Autodesk Inventor part; units mm, degrees
(part 2 of 3)
  spline S35 degree 3 poles (-630.6754, -331.5189) (-629.2902, -331.389) (-626.5198, -331.1292) (-622.3727, -330.655) (-618.2337, -330.1163) (-614.104, -329.509) (-609.9888, -328.8126) (-606.9048, -328.2722) (-604.8663, -327.8241) (-603.9999, -327.726) (-603.303, -327.7315) (-602.786, -327.8061) (-602.2738, -327.9106) (-601.7834, -328.092) (-601.3076, -328.3077) (-600.7153, -328.6749) (-600.1921, -329.1421) (-599.7524, -329.6826) (-599.3924, -330.2793) (-598.9871, -331.0485) (-598.5515, -331.8009) (-598.2378, -332.4231) (-598.014, -333.083) (-597.8968, -333.7746) (-597.901, -334.4715) (-597.9715, -334.9891) (-598.0788, -335.5008) (-598.2628, -335.9901) (-598.4747, -336.4676) (-598.8409, -337.0606) (-599.3849, -337.742) (-600.8488, -339.2296) (-602.9472, -341.5534) (-605.7262, -344.6674) (-608.4377, -347.841) (-611.0958, -351.059) (-613.7038, -354.3181) (-615.3977, -356.5256) (-616.2446, -357.6294) knots 0 0 0 0 0.062506 0.125011 0.187517 0.250023 0.312528 0.375034 0.390661 0.406272 0.414085 0.421898 0.429707 0.43752 0.44533 0.453144 0.468748 0.476562 0.484374 0.5 0.515626 0.523438 0.531252 0.546856 0.55467 0.56248 0.570293 0.578102 0.585915 0.593728 0.609339 0.624966 0.687472 0.749977 0.812483 0.874989 0.937494 1 1 1 1 projected
  arc A39 (-616.2446, -357.6294) -> (-611.0948, -366.3596) centre (0, 0) ccw projected
  spline S36 degree 3 poles (-611.0948, -366.3596) (-609.7191, -366.1523) (-606.9676, -365.7376) (-602.8536, -365.0315) (-598.7514, -364.2616) (-594.6622, -363.4237) (-590.5925, -362.4976) (-587.5436, -361.7852) (-585.5335, -361.2235) (-584.674, -361.077) (-583.9779, -361.0434) (-583.4575, -361.0889) (-582.9402, -361.1645) (-582.4404, -361.3181) (-581.9532, -361.5068) (-581.3414, -361.8402) (-580.7927, -362.2774) (-580.3234, -362.7924) (-579.9306, -363.3679) (-579.4827, -364.1131) (-579.0056, -364.8399) (-578.6575, -365.4436) (-578.3971, -366.0899) (-578.2414, -366.7739) (-578.2064, -367.4699) (-578.2478, -367.9906) (-578.3263, -368.5076) (-578.4825, -369.0064) (-578.6673, -369.495) (-578.9997, -370.1076) (-579.5046, -370.8184) (-580.8828, -372.3858) (-582.8476, -374.8236) (-585.4477, -378.0885) (-587.9769, -381.4091) (-590.4504, -384.7711) (-592.8715, -388.1713) (-594.439, -390.4704) (-595.2227, -391.6199) knots 0 0 0 0 0.062506 0.125011 0.187517 0.250023 0.312528 0.375034 0.390661 0.406272 0.414085 0.421898 0.429707 0.43752 0.44533 0.453144 0.468748 0.476562 0.484374 0.5 0.515626 0.523438 0.531252 0.546856 0.55467 0.56248 0.570293 0.578102 0.585915 0.593728 0.609339 0.624966 0.687472 0.749977 0.812483 0.874989 0.937494 1 1 1 1 projected
  arc A40 (-595.2227, -391.6199) -> (-589.5915, -400.0476) centre (0, 0) ccw projected
  spline S37 degree 3 poles (-589.5915, -400.0476) (-588.2295, -399.7635) (-585.5056, -399.1951) (-581.4377, -398.2595) (-577.3851, -397.2608) (-573.3493, -396.1949) (-569.338, -395.0422) (-566.3339, -394.1599) (-564.3583, -393.4864) (-563.5084, -393.2919) (-562.8153, -393.2193) (-562.2931, -393.2355) (-561.7725, -393.2821) (-561.2648, -393.4074) (-560.7679, -393.5684) (-560.1383, -393.8671) (-559.566, -394.2727) (-559.0685, -394.7606) (-558.644, -395.3133) (-558.1551, -396.0322) (-557.638, -396.7311) (-557.2566, -397.3143) (-556.9604, -397.945) (-556.7665, -398.6191) (-556.6926, -399.312) (-556.7047, -399.8343) (-556.7541, -400.3549) (-556.8821, -400.8617) (-557.0392, -401.3599) (-557.3367, -401.9901) (-557.801, -402.7281) (-559.0892, -404.3703) (-560.9141, -406.9145) (-563.327, -410.32) (-565.6661, -413.7772) (-567.9472, -417.2726) (-570.1739, -420.8032) (-571.61, -423.1866) (-572.328, -424.3782) knots 0 0 0 0 0.062506 0.125011 0.187517 0.250023 0.312528 0.375034 0.390661 0.406272 0.414085 0.421898 0.429707 0.43752 0.44533 0.453144 0.468748 0.476562 0.484374 0.5 0.515626 0.523438 0.531252 0.546856 0.55467 0.56248 0.570293 0.578102 0.585915 0.593728 0.609339 0.624966 0.687472 0.749977 0.812483 0.874989 0.937494 1 1 1 1 projected
  arc A41 (-572.328, -424.3782) -> (-566.2331, -432.4769) centre (0, 0) ccw projected
  spline S38 degree 3 poles (-566.2331, -432.4769) (-564.8892, -432.1169) (-562.2015, -431.3967) (-558.1924, -430.2345) (-554.2022, -429.0101) (-550.2325, -427.7196) (-546.2921, -426.3437) (-543.3422, -425.2944) (-541.4076, -424.5112) (-540.5699, -424.2693) (-539.8819, -424.158) (-539.3597, -424.1449) (-538.8372, -424.1622) (-538.3233, -424.2589) (-537.8181, -424.3918) (-537.1728, -424.6546) (-536.5786, -425.0276) (-536.0546, -425.4868) (-535.5998, -426.0148) (-535.0713, -426.7051) (-534.5159, -427.374) (-534.1023, -427.9349) (-533.7712, -428.5479) (-533.5398, -429.2102) (-533.4272, -429.8979) (-533.41, -430.42) (-533.4301, -430.9425) (-533.5296, -431.4557) (-533.6585, -431.9619) (-533.9201, -432.6078) (-534.3423, -433.3707) (-535.5364, -435.0826) (-537.2158, -437.725) (-539.434, -441.2605) (-541.5755, -444.8434) (-543.6571, -448.4612) (-545.6823, -452.1111) (-546.9825, -454.5712) (-547.6326, -455.8013) knots 0 0 0 0 0.062506 0.125011 0.187517 0.250023 0.312528 0.375034 0.390661 0.406272 0.414085 0.421898 0.429707 0.43752 0.44533 0.453144 0.468748 0.476562 0.484374 0.5 0.515626 0.523438 0.531252 0.546856 0.55467 0.56248 0.570293 0.578102 0.585915 0.593728 0.609339 0.624966 0.687472 0.749977 0.812483 0.874989 0.937494 1 1 1 1 projected
  arc A42 (-547.6326, -455.8013) -> (-541.0931, -463.5455) centre (0, 0) ccw projected
  spline S39 degree 3 poles (-541.0931, -463.5455) (-539.7716, -463.1107) (-537.1284, -462.2409) (-533.1909, -460.8557) (-529.2755, -459.4096) (-525.3845, -457.8985) (-521.5274, -456.3038) (-518.641, -455.0908) (-516.7533, -454.2003) (-515.9305, -453.9119) (-515.2498, -453.7621) (-514.7292, -453.7198) (-514.2066, -453.7077) (-513.6881, -453.7755) (-513.1762, -453.8798) (-512.5171, -454.1061) (-511.903, -454.4451) (-511.354, -454.8742) (-510.8703, -455.3759) (-510.304, -456.0355) (-509.7119, -456.6722) (-509.2676, -457.209) (-508.9026, -457.8025) (-508.6345, -458.4508) (-508.4834, -459.131) (-508.4371, -459.6514) (-508.4278, -460.1742) (-508.4983, -460.6921) (-508.5986, -461.2048) (-508.8237, -461.8644) (-509.2024, -462.6498) (-510.2986, -464.4259) (-511.8272, -467.1583) (-513.8437, -470.8126) (-515.781, -474.51) (-517.6564, -478.2388) (-519.4737, -481.9965) (-520.634, -484.5257) (-521.2141, -485.7902) knots 0 0 0 0 0.062506 0.125011 0.187517 0.250023 0.312528 0.375034 0.390661 0.406272 0.414085 0.421898 0.429707 0.43752 0.44533 0.453144 0.468748 0.476562 0.484374 0.5 0.515626 0.523438 0.531252 0.546856 0.55467 0.56248 0.570293 0.578102 0.585915 0.593728 0.609339 0.624966 0.687472 0.749977 0.812483 0.874989 0.937494 1 1 1 1 projected
  arc A43 (-521.2141, -485.7902) -> (-514.2507, -493.1556) centre (0, 0) ccw projected
  spline S40 degree 3 poles (-514.2507, -493.1556) (-512.9556, -492.6473) (-510.3654, -491.6307) (-506.5117, -490.027) (-502.6836, -488.3636) (-498.8834, -486.6367) (-495.1218, -484.8283) (-492.3079, -483.4553) (-490.4731, -482.4603) (-489.6678, -482.1262) (-488.9966, -481.9385) (-488.4791, -481.8671) (-487.958, -481.8258) (-487.4366, -481.8643) (-486.9196, -481.9398) (-486.2489, -482.1288) (-485.6167, -482.4328) (-485.0446, -482.8305) (-484.5335, -483.3042) (-483.9311, -483.9311) (-483.3042, -484.5335) (-482.8305, -485.0446) (-482.4328, -485.6167) (-482.1288, -486.2489) (-481.9398, -486.9196) (-481.8643, -487.4366) (-481.8258, -487.958) (-481.8671, -488.4791) (-481.9385, -488.9966) (-482.1262, -489.6678) (-482.4603, -490.4731) (-483.4553, -492.3079) (-484.8283, -495.1218) (-486.6367, -498.8834) (-488.3636, -502.6836) (-490.027, -506.5117) (-491.6307, -510.3654) (-492.6473, -512.9556) (-493.1556, -514.2507) knots 0 0 0 0 0.062506 0.125011 0.187517 0.250023 0.312528 0.375034 0.390661 0.406272 0.414085 0.421898 0.429707 0.43752 0.44533 0.453144 0.468748 0.476562 0.484374 0.5 0.515626 0.523438 0.531252 0.546856 0.55467 0.56248 0.570293 0.578102 0.585915 0.593728 0.609339 0.624966 0.687472 0.749977 0.812483 0.874989 0.937494 1 1 1 1 projected
  arc A44 (-493.1556, -514.2507) -> (-485.7902, -521.2141) centre (0, 0) ccw projected
  spline S41 degree 3 poles (-485.7902, -521.2141) (-484.5257, -520.634) (-481.9965, -519.4737) (-478.2388, -517.6564) (-474.51, -515.781) (-470.8126, -513.8437) (-467.1583, -511.8272) (-464.4259, -510.2986) (-462.6498, -509.2024) (-461.8644, -508.8237) (-461.2048, -508.5986) (-460.6921, -508.4983) (-460.1742, -508.4278) (-459.6514, -508.4371) (-459.131, -508.4834) (-458.4508, -508.6345) (-457.8025, -508.9026) (-457.209, -509.2676) (-456.6722, -509.7119) (-456.0355, -510.304) (-455.3759, -510.8703) (-454.8742, -511.354) (-454.4451, -511.903) (-454.1061, -512.5171) (-453.8798, -513.1762) (-453.7755, -513.6881) (-453.7077, -514.2066) (-453.7198, -514.7292) (-453.7621, -515.2498) (-453.9119, -515.9305) (-454.2003, -516.7533) (-455.0908, -518.641) (-456.3038, -521.5274) (-457.8985, -525.3845) (-459.4096, -529.2755) (-460.8557, -533.1909) (-462.2409, -537.1284) (-463.1107, -539.7716) (-463.5455, -541.0931) knots 0 0 0 0 0.062506 0.125011 0.187517 0.250023 0.312528 0.375034 0.390661 0.406272 0.414085 0.421898 0.429707 0.43752 0.44533 0.453144 0.468748 0.476562 0.484374 0.5 0.515626 0.523438 0.531252 0.546856 0.55467 0.56248 0.570293 0.578102 0.585915 0.593728 0.609339 0.624966 0.687472 0.749977 0.812483 0.874989 0.937494 1 1 1 1 projected
  arc A45 (-463.5455, -541.0931) -> (-455.8013, -547.6326) centre (0, 0) ccw projected
  spline S42 degree 3 poles (-455.8013, -547.6326) (-454.5712, -546.9825) (-452.1111, -545.6823) (-448.4612, -543.6571) (-444.8434, -541.5755) (-441.2605, -539.434) (-437.725, -537.2158) (-435.0826, -535.5364) (-433.3707, -534.3423) (-432.6078, -533.9201) (-431.9619, -533.6585) (-431.4557, -533.5296) (-430.9425, -533.4301) (-430.42, -533.41) (-429.8979, -533.4272) (-429.2102, -533.5398) (-428.5479, -533.7712) (-427.9349, -534.1023) (-427.374, -534.5159) (-426.7051, -535.0713) (-426.0148, -535.5998) (-425.4868, -536.0546) (-425.0276, -536.5786) (-424.6546, -537.1728) (-424.3918, -537.8181) (-424.2589, -538.3233) (-424.1622, -538.8372) (-424.1449, -539.3597) (-424.158, -539.8819) (-424.2693, -540.5699) (-424.5112, -541.4076) (-425.2944, -543.3422) (-426.3437, -546.2921) (-427.7196, -550.2325) (-429.0101, -554.2022) (-430.2345, -558.1924) (-431.3967, -562.2015) (-432.1169, -564.8892) (-432.4769, -566.2331) knots 0 0 0 0 0.062506 0.125011 0.187517 0.250023 0.312528 0.375034 0.390661 0.406272 0.414085 0.421898 0.429707 0.43752 0.44533 0.453144 0.468748 0.476562 0.484374 0.5 0.515626 0.523438 0.531252 0.546856 0.55467 0.56248 0.570293 0.578102 0.585915 0.593728 0.609339 0.624966 0.687472 0.749977 0.812483 0.874989 0.937494 1 1 1 1 projected
  arc A46 (-432.4769, -566.2331) -> (-424.3782, -572.328) centre (0, 0) ccw projected
  spline S43 degree 3 poles (-424.3782, -572.328) (-423.1866, -571.61) (-420.8032, -570.1739) (-417.2726, -567.9472) (-413.7772, -565.6661) (-410.32, -563.327) (-406.9145, -560.9141) (-404.3703, -559.0892) (-402.7281, -557.801) (-401.9901, -557.3367) (-401.3599, -557.0392) (-400.8617, -556.8821) (-400.3549, -556.7541) (-399.8343, -556.7047) (-399.312, -556.6926) (-398.6191, -556.7665) (-397.945, -556.9604) (-397.3143, -557.2566) (-396.7311, -557.638) (-396.0322, -558.1551) (-395.3133, -558.644) (-394.7606, -559.0685) (-394.2727, -559.566) (-393.8671, -560.1383) (-393.5684, -560.7679) (-393.4074, -561.2648) (-393.2821, -561.7725) (-393.2355, -562.2931) (-393.2193, -562.8153) (-393.2919, -563.5084) (-393.4864, -564.3583) (-394.1599, -566.3339) (-395.0422, -569.338) (-396.1949, -573.3493) (-397.2608, -577.3851) (-398.2595, -581.4377) (-399.1951, -585.5056) (-399.7635, -588.2295) (-400.0476, -589.5915) knots 0 0 0 0 0.062506 0.125011 0.187517 0.250023 0.312528 0.375034 0.390661 0.406272 0.414085 0.421898 0.429707 0.43752 0.44533 0.453144 0.468748 0.476562 0.484374 0.5 0.515626 0.523438 0.531252 0.546856 0.55467 0.56248 0.570293 0.578102 0.585915 0.593728 0.609339 0.624966 0.687472 0.749977 0.812483 0.874989 0.937494 1 1 1 1 projected
  arc A47 (-400.0476, -589.5915) -> (-391.6199, -595.2227) centre (0, 0) ccw projected
  spline S44 degree 3 poles (-391.6199, -595.2227) (-390.4704, -594.439) (-388.1713, -592.8715) (-384.7711, -590.4504) (-381.4091, -587.9769) (-378.0885, -585.4477) (-374.8236, -582.8476) (-372.3858, -580.8828) (-370.8184, -579.5046) (-370.1076, -578.9997) (-369.495, -578.6673) (-369.0064, -578.4825) (-368.5076, -578.3263) (-367.9906, -578.2478) (-367.4699, -578.2064) (-366.7739, -578.2414) (-366.0899, -578.3971) (-365.4436, -578.6575) (-364.8399, -579.0056) (-364.1131, -579.4827) (-363.3679, -579.9306) (-362.7924, -580.3234) (-362.2774, -580.7927) (-361.8402, -581.3414) (-361.5068, -581.9532) (-361.3181, -582.4404) (-361.1645, -582.9402) (-361.0889, -583.4575) (-361.0434, -583.9779) (-361.077, -584.674) (-361.2235, -585.5335) (-361.7852, -587.5436) (-362.4976, -590.5925) (-363.4237, -594.6622) (-364.2616, -598.7514) (-365.0315, -602.8536) (-365.7376, -606.9676) (-366.1523, -609.7191) (-366.3596, -611.0948) knots 0 0 0 0 0.062506 0.125011 0.187517 0.250023 0.312528 0.375034 0.390661 0.406272 0.414085 0.421898 0.429707 0.43752 0.44533 0.453144 0.468748 0.476562 0.484374 0.5 0.515626 0.523438 0.531252 0.546856 0.55467 0.56248 0.570293 0.578102 0.585915 0.593728 0.609339 0.624966 0.687472 0.749977 0.812483 0.874989 0.937494 1 1 1 1 projected
  arc A48 (-366.3596, -611.0948) -> (-357.6294, -616.2446) centre (0, 0) ccw projected
  spline S45 degree 3 poles (-357.6294, -616.2446) (-356.5256, -615.3977) (-354.3181, -613.7038) (-351.059, -611.0958) (-347.841, -608.4377) (-344.6674, -605.7262) (-341.5534, -602.9472) (-339.2296, -600.8488) (-337.742, -599.3849) (-337.0606, -598.8409) (-336.4676, -598.4747) (-335.9901, -598.2628) (-335.5008, -598.0788) (-334.9891, -597.9715) (-334.4715, -597.901) (-333.7746, -597.8968) (-333.083, -598.014) (-332.4231, -598.2378) (-331.8009, -598.5515) (-331.0485, -598.9871) (-330.2793, -599.3924) (-329.6826, -599.7524) (-329.1421, -600.1921) (-328.6749, -600.7153) (-328.3077, -601.3076) (-328.092, -601.7834) (-327.9106, -602.2738) (-327.8061, -602.786) (-327.7315, -603.303) (-327.726, -603.9999) (-327.8241, -604.8663) (-328.2722, -606.9048) (-328.8126, -609.9888) (-329.509, -614.104) (-330.1163, -618.2337) (-330.655, -622.3727) (-331.1292, -626.5198) (-331.389, -629.2902) (-331.5189, -630.6754) knots 0 0 0 0 0.062506 0.125011 0.187517 0.250023 0.312528 0.375034 0.390661 0.406272 0.414085 0.421898 0.429707 0.43752 0.44533 0.453144 0.468748 0.476562 0.484374 0.5 0.515626 0.523438 0.531252 0.546856 0.55467 0.56248 0.570293 0.578102 0.585915 0.593728 0.609339 0.624966 0.687472 0.749977 0.812483 0.874989 0.937494 1 1 1 1 projected
  arc A49 (-331.5189, -630.6754) -> (-322.5137, -635.3276) centre (0, 0) ccw projected
  spline S46 degree 3 poles (-322.5137, -635.3276) (-321.4591, -634.4201) (-319.35, -632.6051) (-316.2423, -629.8185) (-313.1784, -626.9841) (-310.1618, -624.099) (-307.2086, -621.1497) (-305.0061, -618.9244) (-303.6029, -617.3793) (-302.9531, -616.7979) (-302.3815, -616.3991) (-301.9167, -616.1608) (-301.4385, -615.9496) (-300.9335, -615.8138) (-300.4207, -615.7143) (-299.7252, -615.6711) (-299.0281, -615.7494) (-298.3567, -615.9357) (-297.7178, -616.2141) (-296.9422, -616.6068) (-296.1515, -616.9684) (-295.5356, -617.2943) (-294.9713, -617.703) (-294.4755, -618.1993) (-294.0756, -618.77) (-293.8336, -619.2329) (-293.625, -619.7124) (-293.4919, -620.2179) (-293.3884, -620.73) (-293.3439, -621.4255) (-293.3933, -622.296) (-293.7264, -624.3564) (-294.093, -627.4658) (-294.5575, -631.6136) (-294.9324, -635.7709) (-295.2381, -639.9336) (-295.4791, -644.1007) (-295.5831, -646.8813) (-295.6351, -648.2716) knots 0 0 0 0 0.062506 0.125011 0.187517 0.250023 0.312528 0.375034 0.390661 0.406272 0.414085 0.421898 0.429707 0.43752 0.44533 0.453144 0.468748 0.476562 0.484374 0.5 0.515626 0.523438 0.531252 0.546856 0.55467 0.56248 0.570293 0.578102 0.585915 0.593728 0.609339 0.624966 0.687472 0.749977 0.812483 0.874989 0.937494 1 1 1 1 projected
  arc A50 (-295.6351, -648.2716) -> (-286.3832, -652.4116) centre (0, 0) ccw projected
  spline S47 degree 3 poles (-286.3832, -652.4116) (-285.3812, -651.4464) (-283.3772, -649.5159) (-280.4306, -646.5595) (-277.5304, -643.5578) (-274.6804, -640.508) (-271.8971, -637.3978) (-269.8229, -635.0525) (-268.5085, -633.4312) (-267.8923, -632.8143) (-267.3441, -632.3841) (-266.8933, -632.12) (-266.4277, -631.8824) (-265.9312, -631.7185) (-265.4247, -631.5904) (-264.7327, -631.5083) (-264.0323, -631.5473) (-263.3515, -631.6957) (-262.6981, -631.9378) (-261.9016, -632.2864) (-261.0919, -632.6031) (-260.4587, -632.894) (-259.8724, -633.2704) (-259.3495, -633.7381) (-258.9182, -634.2855) (-258.6507, -634.7342) (-258.4155, -635.2012) (-258.2543, -635.6984) (-258.1223, -636.2039) (-258.0388, -636.8958) (-258.0393, -637.7677) (-258.2563, -639.8435) (-258.448, -642.9686) (-258.6792, -647.1359) (-258.8204, -651.3077) (-258.8923, -655.481) (-258.8992, -659.655) (-258.8472, -662.4371) (-258.8212, -663.8282) knots 0 0 0 0 0.062506 0.125011 0.187517 0.250023 0.312528 0.375034 0.390661 0.406272 0.414085 0.421898 0.429707 0.43752 0.44533 0.453144 0.468748 0.476562 0.484374 0.5 0.515626 0.523438 0.531252 0.546856 0.55467 0.56248 0.570293 0.578102 0.585915 0.593728 0.609339 0.624966 0.687472 0.749977 0.812483 0.874989 0.937494 1 1 1 1 projected
  arc A51 (-258.8212, -663.8282) -> (-249.3517, -667.4429) centre (0, 0) ccw projected
  spline S48 degree 3 poles (-249.3517, -667.4429) (-248.4053, -666.423) (-246.5127, -664.3832) (-243.7365, -661.2662) (-241.0092, -658.1066) (-238.3347, -654.9019) (-235.7302, -651.6405) (-233.7907, -649.1825) (-232.5693, -647.4901) (-231.9887, -646.8396) (-231.4654, -646.3793) (-231.0302, -646.0904) (-230.5786, -645.8271) (-230.0921, -645.6356) (-229.5936, -645.4793) (-228.9073, -645.3585) (-228.2058, -645.3582) (-227.5178, -645.4682) (-226.8518, -645.6733) (-226.037, -645.9767) (-225.2109, -646.2475) (-224.5623, -646.5024) (-223.9558, -646.8453) (-223.4075, -647.2829) (-222.9463, -647.8053) (-222.654, -648.2383) (-222.393, -648.6914) (-222.2041, -649.1788) (-222.044, -649.676) (-221.9218, -650.3622) (-221.8734, -651.2327) (-221.9737, -653.3175) (-221.9899, -656.4484) (-221.9871, -660.6221) (-221.8941, -664.7953) (-221.7319, -668.966) (-221.5048, -673.1339) (-221.2968, -675.9087) (-221.1928, -677.2961) knots 0 0 0 0 0.062506 0.125011 0.187517 0.250023 0.312528 0.375034 0.390661 0.406272 0.414085 0.421898 0.429707 0.43752 0.44533 0.453144 0.468748 0.476562 0.484374 0.5 0.515626 0.523438 0.531252 0.546856 0.55467 0.56248 0.570293 0.578102 0.585915 0.593728 0.609339 0.624966 0.687472 0.749977 0.812483 0.874989 0.937494 1 1 1 1 projected
  arc A52 (-221.1928, -677.2961) -> (-211.5356, -680.3741) centre (0, 0) ccw projected
  spline S49 degree 3 poles (-211.5356, -680.3741) (-210.6479, -679.3028) (-208.8726, -677.1601) (-206.2756, -673.8923) (-203.7298, -670.5848) (-201.2391, -667.2351) (-198.8216, -663.8328) (-197.023, -661.27) (-195.8984, -659.5117) (-195.3552, -658.8297) (-194.8585, -658.3408) (-194.4401, -658.028) (-194.0041, -657.7397) (-193.529, -657.5212) (-193.0401, -657.3372) (-192.3616, -657.1782) (-191.6613, -657.1385) (-190.9681, -657.2098) (-190.2917, -657.3772) (-189.4612, -657.6344) (-188.6212, -657.8585) (-187.9593, -658.0766) (-187.3345, -658.385) (-186.7626, -658.7912) (-186.2728, -659.2869) (-185.9567, -659.7028) (-185.6707, -660.1405) (-185.4548, -660.6166) (-185.267, -661.1041) (-185.1066, -661.7823) (-185.0095, -662.6487) (-184.9927, -664.7358) (-184.8333, -667.8628) (-184.5965, -672.0298) (-184.2697, -676.1911) (-183.8738, -680.3462) (-183.4134, -684.4948) (-183.0502, -687.2536) (-182.8686, -688.6329) knots 0 0 0 0 0.062506 0.125011 0.187517 0.250023 0.312528 0.375034 0.390661 0.406272 0.414085 0.421898 0.429707 0.43752 0.44533 0.453144 0.468748 0.476562 0.484374 0.5 0.515626 0.523438 0.531252 0.546856 0.55467 0.56248 0.570293 0.578102 0.585915 0.593728 0.609339 0.624966 0.687472 0.749977 0.812483 0.874989 0.937494 1 1 1 1 projected
  arc A53 (-182.8686, -688.6329) -> (-173.0539, -691.1647) centre (0, 0) ccw projected
  spline S50 degree 3 poles (-173.0539, -691.1647) (-172.2277, -690.0452) (-170.5754, -687.8064) (-168.1656, -684.3981) (-165.8093, -680.953) (-163.5103, -677.469) (-161.2874, -673.9365) (-159.6353, -671.2769) (-158.6111, -669.4583) (-158.1069, -668.7469) (-157.6385, -668.2309) (-157.2383, -667.8951) (-156.8191, -667.5829) (-156.357, -667.3381) (-155.8792, -667.127) (-155.2107, -666.9301) (-154.5137, -666.8512) (-153.8177, -666.8835) (-153.1329, -667.0128) (-152.2893, -667.223) (-151.438, -667.3996) (-150.765, -667.5803) (-150.1239, -667.8532) (-149.5301, -668.2267) (-149.0132, -668.6941) (-148.6743, -669.0916) (-148.3642, -669.5126) (-148.122, -669.9759) (-147.9072, -670.452) (-147.709, -671.1202) (-147.5634, -671.9798) (-147.4297, -674.0627) (-147.0952, -677.1758) (-146.6251, -681.3229) (-146.0655, -685.4594) (-145.4372, -689.5858) (-144.7449, -693.702) (-144.2276, -696.4361) (-143.9689, -697.8031) knots 0 0 0 0 0.062506 0.125011 0.187517 0.250023 0.312528 0.375034 0.390661 0.406272 0.414085 0.421898 0.429707 0.43752 0.44533 0.453144 0.468748 0.476562 0.484374 0.5 0.515626 0.523438 0.531252 0.546856 0.55467 0.56248 0.570293 0.578102 0.585915 0.593728 0.609339 0.624966 0.687472 0.749977 0.812483 0.874989 0.937494 1 1 1 1 projected
  arc A54 (-143.9689, -697.8031) -> (-134.0277, -699.7805) centre (0, 0) ccw projected
  spline S51 degree 3 poles (-134.0277, -699.7805) (-133.2656, -698.6166) (-131.7414, -696.2886) (-129.5266, -692.7506) (-127.3671, -689.1788) (-125.2671, -685.5713) (-123.2458, -681.9197) (-121.7454, -679.1716) (-120.8247, -677.2985) (-120.3613, -676.56) (-119.9225, -676.0185) (-119.5418, -675.6608) (-119.1407, -675.3255) (-118.6931, -675.0552) (-118.2279, -674.8177) (-117.5715, -674.5836) (-116.88, -674.4658) (-116.1832, -674.459) (-115.4923, -674.5497) (-114.6382, -674.7123) (-113.7784, -674.8409) (-113.0963, -674.9835) (-112.4409, -675.22) (-111.8271, -675.5596) (-111.2848, -675.9973) (-110.9241, -676.3752) (-110.5909, -676.7782) (-110.3231, -677.2271) (-110.0819, -677.6905) (-109.8466, -678.3465) (-109.6531, -679.1966) (-109.4027, -681.2687) (-108.8942, -684.3582) (-108.1923, -688.4724) (-107.4016, -692.571) (-106.5431, -696.6556) (-105.621, -700.7266) (-104.9512, -703.4274) (-104.6163, -704.7778) knots 0 0 0 0 0.062506 0.125011 0.187517 0.250023 0.312528 0.375034 0.390661 0.406272 0.414085 0.421898 0.429707 0.43752 0.44533 0.453144 0.468748 0.476562 0.484374 0.5 0.515626 0.523438 0.531252 0.546856 0.55467 0.56248 0.570293 0.578102 0.585915 0.593728 0.609339 0.624966 0.687472 0.749977 0.812483 0.874989 0.937494 1 1 1 1 projected
  arc A55 (-104.6163, -704.7778) -> (-94.5799, -706.1947) centre (0, 0) ccw projected
  spline S52 degree 3 poles (-94.5799, -706.1947) (-93.8842, -704.9898) (-92.4929, -702.58) (-90.48, -698.9234) (-88.5241, -695.2361) (-86.6297, -691.5166) (-84.8163, -687.7574) (-83.4724, -684.9295) (-82.6582, -683.0077) (-82.2369, -682.2443) (-81.8292, -681.6791) (-81.4691, -681.3006) (-81.0875, -680.9434) (-80.6558, -680.6484) (-80.2045, -680.3852) (-79.5623, -680.1147) (-78.8785, -679.9583) (-78.1832, -679.9124) (-77.4883, -679.9642) (-76.6265, -680.0787) (-75.7608, -680.1588) (-75.0717, -680.263) (-74.4041, -680.4624) (-73.7722, -680.7671) (-73.2063, -681.1737) (-72.825, -681.5307) (-72.4697, -681.9144) (-72.1771, -682.3476) (-71.9103, -682.7967) (-71.6386, -683.4385) (-71.3977, -684.2764) (-71.0316, -686.3312) (-70.3506, -689.3873) (-69.4192, -693.4557) (-68.3999, -697.5035) (-67.3136, -701.5336) (-66.1648, -705.5465) (-65.3446, -708.2054) (-64.9345, -709.5349) knots 0 0 0 0 0.062506 0.125011 0.187517 0.250023 0.312528 0.375034 0.390661 0.406272 0.414085 0.421898 0.429707 0.43752 0.44533 0.453144 0.468748 0.476562 0.484374 0.5 0.515626 0.523438 0.531252 0.546856 0.55467 0.56248 0.570293 0.578102 0.585915 0.593728 0.609339 0.624966 0.687472 0.749977 0.812483 0.874989 0.937494 1 1 1 1 projected
  arc A56 (-64.9345, -709.5349) -> (-54.8344, -710.3868) centre (0, 0) ccw projected
  spline S53 degree 3 poles (-54.8344, -710.3868) (-54.2075, -709.1448) (-52.9535, -706.6608) (-51.1487, -702.8971) (-49.4027, -699.1059) (-47.7198, -695.286) (-46.12, -691.4311) (-44.9368, -688.5323) (-44.2317, -686.5679) (-43.8538, -685.7821) (-43.4784, -685.1949) (-43.1401, -684.7968) (-42.7791, -684.4188) (-42.3646, -684.1) (-41.9289, -683.8119) (-41.3028, -683.5058) (-40.6288, -683.3113) (-39.9372, -683.2266) (-39.2405, -683.2393) (-38.3736, -683.3053) (-37.5048, -683.3367) (-36.811, -683.4021) (-36.1332, -683.5638) (-35.4853, -683.8325) (-34.8974, -684.2068) (-34.4967, -684.5419) (-34.1205, -684.905) (-33.8041, -685.3211) (-33.5125, -685.7546) (-33.2052, -686.3801) (-32.9177, -687.2032) (-32.4369, -689.2343) (-31.5857, -692.2473) (-30.4276, -696.2572) (-29.183, -700.2414) (-27.8724, -704.2043) (-26.5004, -708.1464) (-25.5324, -710.7552) (-25.0484, -712.0596) knots 0 0 0 0 0.062506 0.125011 0.187517 0.250023 0.312528 0.375034 0.390661 0.406272 0.414085 0.421898 0.429707 0.43752 0.44533 0.453144 0.468748 0.476562 0.484374 0.5 0.515626 0.523438 0.531252 0.546856 0.55467 0.56248 0.570293 0.578102 0.585915 0.593728 0.609339 0.624966 0.687472 0.749977 0.812483 0.874989 0.937494 1 1 1 1 projected
  arc A57 (-25.0484, -712.0596) -> (-14.9165, -712.3438) centre (0, 0) ccw projected
  spline S54 degree 3 poles (-14.9165, -712.3438) (-14.3601, -711.0686) (-13.2474, -708.5182) (-11.6564, -704.6592) (-10.1258, -700.7761) (-8.6597, -696.8679) (-7.2786, -692.9293) (-6.2598, -689.9687) (-5.6659, -687.9678) (-5.3327, -687.1621) (-4.9908, -686.5548) (-4.6754, -686.1384) (-4.3362, -685.7407) (-3.9402, -685.3992) (-3.5213, -685.0871) (-2.9134, -684.7464) (-2.2513, -684.5144) (-1.5656, -684.391) (-0.8692, -684.3646) (0, -684.3819) (0.8692, -684.3646) (1.5656, -684.391) (2.2513, -684.5144) (2.9134, -684.7464) (3.5213, -685.0871) (3.9402, -685.3992) (4.3362, -685.7407) (4.6754, -686.1384) (4.9908, -686.5548) (5.3327, -687.1621) (5.6659, -687.9678) (6.2598, -689.9687) (7.2786, -692.9293) (8.6597, -696.8679) (10.1258, -700.7761) (11.6564, -704.6592) (13.2474, -708.5182) (14.3601, -711.0686) (14.9165, -712.3438) knots 0 0 0 0 0.062506 0.125011 0.187517 0.250023 0.312528 0.375034 0.390661 0.406272 0.414085 0.421898 0.429707 0.43752 0.44533 0.453144 0.468748 0.476562 0.484374 0.5 0.515626 0.523438 0.531252 0.546856 0.55467 0.56248 0.570293 0.578102 0.585915 0.593728 0.609339 0.624966 0.687472 0.749977 0.812483 0.874989 0.937494 1 1 1 1 projected
  arc A58 (14.9165, -712.3438) -> (25.0484, -712.0596) centre (0, 0) ccw projected
  spline S55 degree 3 poles (25.0484, -712.0596) (25.5324, -710.7552) (26.5004, -708.1464) (27.8724, -704.2043) (29.183, -700.2414) (30.4276, -696.2572) (31.5857, -692.2473) (32.4369, -689.2343) (32.9177, -687.2032) (33.2052, -686.3801) (33.5125, -685.7546) (33.8041, -685.3211) (34.1205, -684.905) (34.4967, -684.5419) (34.8974, -684.2068) (35.4853, -683.8325) (36.1332, -683.5638) (36.811, -683.4021) (37.5048, -683.3367) (38.3736, -683.3053) (39.2405, -683.2393) (39.9372, -683.2266) (40.6288, -683.3113) (41.3028, -683.5058) (41.9289, -683.8119) (42.3646, -684.1) (42.7791, -684.4188) (43.1401, -684.7968) (43.4784, -685.1949) (43.8538, -685.7821) (44.2317, -686.5679) (44.9368, -688.5323) (46.12, -691.4311) (47.7198, -695.286) (49.4027, -699.1059) (51.1487, -702.8971) (52.9535, -706.6608) (54.2075, -709.1448) (54.8344, -710.3868) knots 0 0 0 0 0.062506 0.125011 0.187517 0.250023 0.312528 0.375034 0.390661 0.406272 0.414085 0.421898 0.429707 0.43752 0.44533 0.453144 0.468748 0.476562 0.484374 0.5 0.515626 0.523438 0.531252 0.546856 0.55467 0.56248 0.570293 0.578102 0.585915 0.593728 0.609339 0.624966 0.687472 0.749977 0.812483 0.874989 0.937494 1 1 1 1 projected
  arc A59 (54.8344, -710.3868) -> (64.9345, -709.5349) centre (0, 0) ccw projected
  spline S56 degree 3 poles (64.9345, -709.5349) (65.3446, -708.2054) (66.1648, -705.5465) (67.3136, -701.5336) (68.3999, -697.5035) (69.4192, -693.4557) (70.3506, -689.3873) (71.0316, -686.3312) (71.3977, -684.2764) (71.6386, -683.4385) (71.9103, -682.7967) (72.1771, -682.3476) (72.4697, -681.9144) (72.825, -681.5307) (73.2063, -681.1737) (73.7722, -680.7671) (74.4041, -680.4624) (75.0717, -680.263) (75.7608, -680.1588) (76.6265, -680.0787) (77.4883, -679.9642) (78.1832, -679.9124) (78.8785, -679.9583) (79.5623, -680.1147) (80.2045, -680.3852) (80.6558, -680.6484) (81.0875, -680.9434) (81.4691, -681.3006) (81.8292, -681.6791) (82.2369, -682.2443) (82.6582, -683.0077) (83.4724, -684.9295) (84.8163, -687.7574) (86.6297, -691.5166) (88.5241, -695.2361) (90.48, -698.9234) (92.4929, -702.58) (93.8842, -704.9898) (94.5799, -706.1947) knots 0 0 0 0 0.062506 0.125011 0.187517 0.250023 0.312528 0.375034 0.390661 0.406272 0.414085 0.421898 0.429707 0.43752 0.44533 0.453144 0.468748 0.476562 0.484374 0.5 0.515626 0.523438 0.531252 0.546856 0.55467 0.56248 0.570293 0.578102 0.585915 0.593728 0.609339 0.624966 0.687472 0.749977 0.812483 0.874989 0.937494 1 1 1 1 projected
  arc A60 (94.5799, -706.1947) -> (104.6163, -704.7778) centre (0, 0) ccw projected
  spline S57 degree 3 poles (104.6163, -704.7778) (104.9512, -703.4274) (105.621, -700.7266) (106.5431, -696.6556) (107.4016, -692.571) (108.1923, -688.4724) (108.8942, -684.3582) (109.4027, -681.2687) (109.6531, -679.1966) (109.8466, -678.3465) (110.0819, -677.6905) (110.3231, -677.2271) (110.5909, -676.7782) (110.9241, -676.3752) (111.2848, -675.9973) (111.8271, -675.5596) (112.4409, -675.22) (113.0963, -674.9835) (113.7784, -674.8409) (114.6382, -674.7123) (115.4923, -674.5497) (116.1832, -674.459) (116.88, -674.4658) (117.5715, -674.5836) (118.2279, -674.8177) (118.6931, -675.0552) (119.1407, -675.3255) (119.5418, -675.6608) (119.9225, -676.0185) (120.3613, -676.56) (120.8247, -677.2985) (121.7454, -679.1716) (123.2458, -681.9197) (125.2671, -685.5713) (127.3671, -689.1788) (129.5266, -692.7506) (131.7414, -696.2886) (133.2656, -698.6166) (134.0277, -699.7805) knots 0 0 0 0 0.062506 0.125011 0.187517 0.250023 0.312528 0.375034 0.390661 0.406272 0.414085 0.421898 0.429707 0.43752 0.44533 0.453144 0.468748 0.476562 0.484374 0.5 0.515626 0.523438 0.531252 0.546856 0.55467 0.56248 0.570293 0.578102 0.585915 0.593728 0.609339 0.624966 0.687472 0.749977 0.812483 0.874989 0.937494 1 1 1 1 projected
  arc A61 (134.0277, -699.7805) -> (143.9689, -697.8031) centre (0, 0) ccw projected
  spline S58 degree 3 poles (143.9689, -697.8031) (144.2276, -696.4361) (144.7449, -693.702) (145.4372, -689.5858) (146.0655, -685.4594) (146.6251, -681.3229) (147.0952, -677.1758) (147.4297, -674.0627) (147.5634, -671.9798) (147.709, -671.1202) (147.9072, -670.452) (148.122, -669.9759) (148.3642, -669.5126) (148.6743, -669.0916) (149.0132, -668.6941) (149.5301, -668.2267) (150.1239, -667.8532) (150.765, -667.5803) (151.438, -667.3996) (152.2893, -667.223) (153.1329, -667.0128) (153.8177, -666.8835) (154.5137, -666.8512) (155.2107, -666.9301) (155.8792, -667.127) (156.357, -667.3381) (156.8191, -667.5829) (157.2383, -667.8951) (157.6385, -668.2309) (158.1069, -668.7469) (158.6111, -669.4583) (159.6353, -671.2769) (161.2874, -673.9365) (163.5103, -677.469) (165.8093, -680.953) (168.1656, -684.3981) (170.5754, -687.8064) (172.2277, -690.0452) (173.0539, -691.1647) knots 0 0 0 0 0.062506 0.125011 0.187517 0.250023 0.312528 0.375034 0.390661 0.406272 0.414085 0.421898 0.429707 0.43752 0.44533 0.453144 0.468748 0.476562 0.484374 0.5 0.515626 0.523438 0.531252 0.546856 0.55467 0.56248 0.570293 0.578102 0.585915 0.593728 0.609339 0.624966 0.687472 0.749977 0.812483 0.874989 0.937494 1 1 1 1 projected
  arc A62 (173.0539, -691.1647) -> (182.8686, -688.6329) centre (0, 0) ccw projected
  spline S59 degree 3 poles (182.8686, -688.6329) (183.0502, -687.2536) (183.4134, -684.4948) (183.8738, -680.3462) (184.2697, -676.1911) (184.5965, -672.0298) (184.8333, -667.8628) (184.9927, -664.7358) (185.0095, -662.6487) (185.1066, -661.7823) (185.267, -661.1041) (185.4548, -660.6166) (185.6707, -660.1405) (185.9567, -659.7028) (186.2728, -659.2869) (186.7626, -658.7912) (187.3345, -658.385) (187.9593, -658.0766) (188.6212, -657.8585) (189.4612, -657.6344) (190.2917, -657.3772) (190.9681, -657.2098) (191.6613, -657.1385) (192.3616, -657.1782) (193.0401, -657.3372) (193.529, -657.5212) (194.0041, -657.7397) (194.4401, -658.028) (194.8585, -658.3408) (195.3552, -658.8297) (195.8984, -659.5117) (197.023, -661.27) (198.8216, -663.8328) (201.2391, -667.2351) (203.7298, -670.5848) (206.2756, -673.8923) (208.8726, -677.1601) (210.6479, -679.3028) (211.5356, -680.3741) knots 0 0 0 0 0.062506 0.125011 0.187517 0.250023 0.312528 0.375034 0.390661 0.406272 0.414085 0.421898 0.429707 0.43752 0.44533 0.453144 0.468748 0.476562 0.484374 0.5 0.515626 0.523438 0.531252 0.546856 0.55467 0.56248 0.570293 0.578102 0.585915 0.593728 0.609339 0.624966 0.687472 0.749977 0.812483 0.874989 0.937494 1 1 1 1 projected
  arc A63 (211.5356, -680.3741) -> (221.1928, -677.2961) centre (0, 0) ccw projected
  spline S60 degree 3 poles (221.1928, -677.2961) (221.2968, -675.9087) (221.5048, -673.1339) (221.7319, -668.966) (221.8941, -664.7953) (221.9871, -660.6221) (221.9899, -656.4484) (221.9737, -653.3175) (221.8734, -651.2327) (221.9218, -650.3622) (222.044, -649.676) (222.2041, -649.1788) (222.393, -648.6914) (222.654, -648.2383) (222.9463, -647.8053) (223.4075, -647.2829) (223.9558, -646.8453) (224.5623, -646.5024) (225.2109, -646.2475) (226.037, -645.9767) (226.8518, -645.6733) (227.5178, -645.4682) (228.2058, -645.3582) (228.9073, -645.3585) (229.5936, -645.4793) (230.0921, -645.6356) (230.5786, -645.8271) (231.0302, -646.0904) (231.4654, -646.3793) (231.9887, -646.8396) (232.5693, -647.4901) (233.7907, -649.1825) (235.7302, -651.6405) (238.3347, -654.9019) (241.0092, -658.1066) (243.7365, -661.2662) (246.5127, -664.3832) (248.4053, -666.423) (249.3517, -667.4429) knots 0 0 0 0 0.062506 0.125011 0.187517 0.250023 0.312528 0.375034 0.390661 0.406272 0.414085 0.421898 0.429707 0.43752 0.44533 0.453144 0.468748 0.476562 0.484374 0.5 0.515626 0.523438 0.531252 0.546856 0.55467 0.56248 0.570293 0.578102 0.585915 0.593728 0.609339 0.624966 0.687472 0.749977 0.812483 0.874989 0.937494 1 1 1 1 projected
  arc A64 (249.3517, -667.4429) -> (258.8212, -663.8282) centre (0, 0) ccw projected
  spline S61 degree 3 poles (258.8212, -663.8282) (258.8472, -662.4371) (258.8992, -659.655) (258.8923, -655.481) (258.8204, -651.3077) (258.6792, -647.1359) (258.448, -642.9686) (258.2563, -639.8435) (258.0393, -637.7677) (258.0388, -636.8958) (258.1223, -636.2039) (258.2543, -635.6984) (258.4155, -635.2012) (258.6507, -634.7342) (258.9182, -634.2855) (259.3495, -633.7381) (259.8724, -633.2704) (260.4587, -632.894) (261.0919, -632.6031) (261.9016, -632.2864) (262.6981, -631.9378) (263.3515, -631.6957) (264.0323, -631.5473) (264.7327, -631.5083) (265.4247, -631.5904) (265.9312, -631.7185) (266.4277, -631.8824) (266.8933, -632.12) (267.3441, -632.3841) (267.8923, -632.8143) (268.5085, -633.4312) (269.8229, -635.0525) (271.8971, -637.3978) (274.6804, -640.508) (277.5304, -643.5578) (280.4306, -646.5595) (283.3772, -649.5159) (285.3812, -651.4464) (286.3832, -652.4116) knots 0 0 0 0 0.062506 0.125011 0.187517 0.250023 0.312528 0.375034 0.390661 0.406272 0.414085 0.421898 0.429707 0.43752 0.44533 0.453144 0.468748 0.476562 0.484374 0.5 0.515626 0.523438 0.531252 0.546856 0.55467 0.56248 0.570293 0.578102 0.585915 0.593728 0.609339 0.624966 0.687472 0.749977 0.812483 0.874989 0.937494 1 1 1 1 projected
  arc A65 (286.3832, -652.4116) -> (295.6351, -648.2716) centre (0, 0) ccw projected
  spline S62 degree 3 poles (295.6351, -648.2716) (295.5831, -646.8813) (295.4791, -644.1007) (295.2381, -639.9336) (294.9324, -635.7709) (294.5575, -631.6136) (294.093, -627.4658) (293.7264, -624.3564) (293.3933, -622.296) (293.3439, -621.4255) (293.3884, -620.73) (293.4919, -620.2179) (293.625, -619.7124) (293.8336, -619.2329) (294.0756, -618.77) (294.4755, -618.1993) (294.9713, -617.703) (295.5356, -617.2943) (296.1515, -616.9684) (296.9422, -616.6068) (297.7178, -616.2141) (298.3567, -615.9357) (299.0281, -615.7494) (299.7252, -615.6711) (300.4207, -615.7143) (300.9335, -615.8138) (301.4385, -615.9496) (301.9167, -616.1608) (302.3815, -616.3991) (302.9531, -616.7979) (303.6029, -617.3793) (305.0061, -618.9244) (307.2086, -621.1497) (310.1618, -624.099) (313.1784, -626.9841) (316.2423, -629.8185) (319.35, -632.6051) (321.4591, -634.4201) (322.5137, -635.3276) knots 0 0 0 0 0.062506 0.125011 0.187517 0.250023 0.312528 0.375034 0.390661 0.406272 0.414085 0.421898 0.429707 0.43752 0.44533 0.453144 0.468748 0.476562 0.484374 0.5 0.515626 0.523438 0.531252 0.546856 0.55467 0.56248 0.570293 0.578102 0.585915 0.593728 0.609339 0.624966 0.687472 0.749977 0.812483 0.874989 0.937494 1 1 1 1 projected
  arc A66 (322.5137, -635.3276) -> (331.5189, -630.6754) centre (0, 0) ccw projected
  spline S63 degree 3 poles (331.5189, -630.6754) (331.389, -629.2902) (331.1292, -626.5198) (330.655, -622.3727) (330.1163, -618.2337) (329.509, -614.104) (328.8126, -609.9888) (328.2722, -606.9048) (327.8241, -604.8663) (327.726, -603.9999) (327.7315, -603.303) (327.8061, -602.786) (327.9106, -602.2738) (328.092, -601.7834) (328.3077, -601.3076) (328.6749, -600.7153) (329.1421, -600.1921) (329.6826, -599.7524) (330.2793, -599.3924) (331.0485, -598.9871) (331.8009, -598.5515) (332.4231, -598.2378) (333.083, -598.014) (333.7746, -597.8968) (334.4715, -597.901) (334.9891, -597.9715) (335.5008, -598.0788) (335.9901, -598.2628) (336.4676, -598.4747) (337.0606, -598.8409) (337.742, -599.3849) (339.2296, -600.8488) (341.5534, -602.9472) (344.6674, -605.7262) (347.841, -608.4377) (351.059, -611.0958) (354.3181, -613.7038) (356.5256, -615.3977) (357.6294, -616.2446) knots 0 0 0 0 0.062506 0.125011 0.187517 0.250023 0.312528 0.375034 0.390661 0.406272 0.414085 0.421898 0.429707 0.43752 0.44533 0.453144 0.468748 0.476562 0.484374 0.5 0.515626 0.523438 0.531252 0.546856 0.55467 0.56248 0.570293 0.578102 0.585915 0.593728 0.609339 0.624966 0.687472 0.749977 0.812483 0.874989 0.937494 1 1 1 1 projected
  arc A67 (357.6294, -616.2446) -> (366.3596, -611.0948) centre (0, 0) ccw projected
  spline S64 degree 3 poles (366.3596, -611.0948) (366.1523, -609.7191) (365.7376, -606.9676) (365.0315, -602.8536) (364.2616, -598.7514) (363.4237, -594.6622) (362.4976, -590.5925) (361.7852, -587.5436) (361.2235, -585.5335) (361.077, -584.674) (361.0434, -583.9779) (361.0889, -583.4575) (361.1645, -582.9402) (361.3181, -582.4404) (361.5068, -581.9532) (361.8402, -581.3414) (362.2774, -580.7927) (362.7924, -580.3234) (363.3679, -579.9306) (364.1131, -579.4827) (364.8399, -579.0056) (365.4436, -578.6575) (366.0899, -578.3971) (366.7739, -578.2414) (367.4699, -578.2064) (367.9906, -578.2478) (368.5076, -578.3263) (369.0064, -578.4825) (369.495, -578.6673) (370.1076, -578.9997) (370.8184, -579.5046) (372.3858, -580.8828) (374.8236, -582.8476) (378.0885, -585.4477) (381.4091, -587.9769) (384.7711, -590.4504) (388.1713, -592.8715) (390.4704, -594.439) (391.6199, -595.2227) knots 0 0 0 0 0.062506 0.125011 0.187517 0.250023 0.312528 0.375034 0.390661 0.406272 0.414085 0.421898 0.429707 0.43752 0.44533 0.453144 0.468748 0.476562 0.484374 0.5 0.515626 0.523438 0.531252 0.546856 0.55467 0.56248 0.570293 0.578102 0.585915 0.593728 0.609339 0.624966 0.687472 0.749977 0.812483 0.874989 0.937494 1 1 1 1 projected
  arc A68 (391.6199, -595.2227) -> (400.0476, -589.5915) centre (0, 0) ccw projected
  spline S65 degree 3 poles (400.0476, -589.5915) (399.7635, -588.2295) (399.1951, -585.5056) (398.2595, -581.4377) (397.2608, -577.3851) (396.1949, -573.3493) (395.0422, -569.338) (394.1599, -566.3339) (393.4864, -564.3583) (393.2919, -563.5084) (393.2193, -562.8153) (393.2355, -562.2931) (393.2821, -561.7725) (393.4074, -561.2648) (393.5684, -560.7679) (393.8671, -560.1383) (394.2727, -559.566) (394.7606, -559.0685) (395.3133, -558.644) (396.0322, -558.1551) (396.7311, -557.638) (397.3143, -557.2566) (397.945, -556.9604) (398.6191, -556.7665) (399.312, -556.6926) (399.8343, -556.7047) (400.3549, -556.7541) (400.8617, -556.8821) (401.3599, -557.0392) (401.9901, -557.3367) (402.7281, -557.801) (404.3703, -559.0892) (406.9145, -560.9141) (410.32, -563.327) (413.7772, -565.6661) (417.2726, -567.9472) (420.8032, -570.1739) (423.1866, -571.61) (424.3782, -572.328) knots 0 0 0 0 0.062506 0.125011 0.187517 0.250023 0.312528 0.375034 0.390661 0.406272 0.414085 0.421898 0.429707 0.43752 0.44533 0.453144 0.468748 0.476562 0.484374 0.5 0.515626 0.523438 0.531252 0.546856 0.55467 0.56248 0.570293 0.578102 0.585915 0.593728 0.609339 0.624966 0.687472 0.749977 0.812483 0.874989 0.937494 1 1 1 1 projected
  arc A69 (424.3782, -572.328) -> (432.4769, -566.2331) centre (0, 0) ccw projected
  spline S66 degree 3 poles (432.4769, -566.2331) (432.1169, -564.8892) (431.3967, -562.2015) (430.2345, -558.1924) (429.0101, -554.2022) (427.7196, -550.2325) (426.3437, -546.2921) (425.2944, -543.3422) (424.5112, -541.4076) (424.2693, -540.5699) (424.158, -539.8819) (424.1449, -539.3597) (424.1622, -538.8372) (424.2589, -538.3233) (424.3918, -537.8181) (424.6546, -537.1728) (425.0276, -536.5786) (425.4868, -536.0546) (426.0148, -535.5998) (426.7051, -535.0713) (427.374, -534.5159) (427.9349, -534.1023) (428.5479, -533.7712) (429.2102, -533.5398) (429.8979, -533.4272) (430.42, -533.41) (430.9425, -533.4301) (431.4557, -533.5296) (431.9619, -533.6585) (432.6078, -533.9201) (433.3707, -534.3423) (435.0826, -535.5364) (437.725, -537.2158) (441.2605, -539.434) (444.8434, -541.5755) (448.4612, -543.6571) (452.1111, -545.6823) (454.5712, -546.9825) (455.8013, -547.6326) knots 0 0 0 0 0.062506 0.125011 0.187517 0.250023 0.312528 0.375034 0.390661 0.406272 0.414085 0.421898 0.429707 0.43752 0.44533 0.453144 0.468748 0.476562 0.484374 0.5 0.515626 0.523438 0.531252 0.546856 0.55467 0.56248 0.570293 0.578102 0.585915 0.593728 0.609339 0.624966 0.687472 0.749977 0.812483 0.874989 0.937494 1 1 1 1 projected
  arc A70 (455.8013, -547.6326) -> (463.5455, -541.0931) centre (0, 0) ccw projected
  spline S67 degree 3 poles (463.5455, -541.0931) (463.1107, -539.7716) (462.2409, -537.1284) (460.8557, -533.1909) (459.4096, -529.2755) (457.8985, -525.3845) (456.3038, -521.5274) (455.0908, -518.641) (454.2003, -516.7533) (453.9119, -515.9305) (453.7621, -515.2498) (453.7198, -514.7292) (453.7077, -514.2066) (453.7755, -513.6881) (453.8798, -513.1762) (454.1061, -512.5171) (454.4451, -511.903) (454.8742, -511.354) (455.3759, -510.8703) (456.0355, -510.304) (456.6722, -509.7119) (457.209, -509.2676) (457.8025, -508.9026) (458.4508, -508.6345) (459.131, -508.4834) (459.6514, -508.4371) (460.1742, -508.4278) (460.6921, -508.4983) (461.2048, -508.5986) (461.8644, -508.8237) (462.6498, -509.2024) (464.4259, -510.2986) (467.1583, -511.8272) (470.8126, -513.8437) (474.51, -515.781) (478.2388, -517.6564) (481.9965, -519.4737) (484.5257, -520.634) (485.7902, -521.2141) knots 0 0 0 0 0.062506 0.125011 0.187517 0.250023 0.312528 0.375034 0.390661 0.406272 0.414085 0.421898 0.429707 0.43752 0.44533 0.453144 0.468748 0.476562 0.484374 0.5 0.515626 0.523438 0.531252 0.546856 0.55467 0.56248 0.570293 0.578102 0.585915 0.593728 0.609339 0.624966 0.687472 0.749977 0.812483 0.874989 0.937494 1 1 1 1 projected
  arc A71 (485.7902, -521.2141) -> (493.1556, -514.2507) centre (0, 0) ccw projected
  spline S68 degree 3 poles (493.1556, -514.2507) (492.6473, -512.9556) (491.6307, -510.3654) (490.027, -506.5117) (488.3636, -502.6836) (486.6367, -498.8834) (484.8283, -495.1218) (483.4553, -492.3079) (482.4603, -490.4731) (482.1262, -489.6678) (481.9385, -488.9966) (481.8671, -488.4791) (481.8258, -487.958) (481.8643, -487.4366) (481.9398, -486.9196) (482.1288, -486.2489) (482.4328, -485.6167) (482.8305, -485.0446) (483.3042, -484.5335) (483.9311, -483.9311) (484.5335, -483.3042) (485.0446, -482.8305) (485.6167, -482.4328) (486.2489, -482.1288) (486.9196, -481.9398) (487.4366, -481.8643) (487.958, -481.8258) (488.4791, -481.8671) (488.9966, -481.9385) (489.6678, -482.1262) (490.4731, -482.4603) (492.3079, -483.4553) (495.1218, -484.8283) (498.8834, -486.6367) (502.6836, -488.3636) (506.5117, -490.027) (510.3654, -491.6307) (512.9556, -492.6473) (514.2507, -493.1556) knots 0 0 0 0 0.062506 0.125011 0.187517 0.250023 0.312528 0.375034 0.390661 0.406272 0.414085 0.421898 0.429707 0.43752 0.44533 0.453144 0.468748 0.476562 0.484374 0.5 0.515626 0.523438 0.531252 0.546856 0.55467 0.56248 0.570293 0.578102 0.585915 0.593728 0.609339 0.624966 0.687472 0.749977 0.812483 0.874989 0.937494 1 1 1 1 projected
  arc A72 (514.2507, -493.1556) -> (521.2141, -485.7902) centre (0, 0) ccw projected
  spline S69 degree 3 poles (521.2141, -485.7902) (520.634, -484.5257) (519.4737, -481.9965) (517.6564, -478.2388) (515.781, -474.51) (513.8437, -470.8126) (511.8272, -467.1583) (510.2986, -464.4259) (509.2024, -462.6498) (508.8237, -461.8644) (508.5986, -461.2048) (508.4983, -460.6921) (508.4278, -460.1742) (508.4371, -459.6514) (508.4834, -459.131) (508.6345, -458.4508) (508.9026, -457.8025) (509.2676, -457.209) (509.7119, -456.6722) (510.304, -456.0355) (510.8703, -455.3759) (511.354, -454.8742) (511.903, -454.4451) (512.5171, -454.1061) (513.1762, -453.8798) (513.6881, -453.7755) (514.2066, -453.7077) (514.7292, -453.7198) (515.2498, -453.7621) (515.9305, -453.9119) (516.7533, -454.2003) (518.641, -455.0908) (521.5274, -456.3038) (525.3845, -457.8985) (529.2755, -459.4096) (533.1909, -460.8557) (537.1284, -462.2409) (539.7716, -463.1107) (541.0931, -463.5455) knots 0 0 0 0 0.062506 0.125011 0.187517 0.250023 0.312528 0.375034 0.390661 0.406272 0.414085 0.421898 0.429707 0.43752 0.44533 0.453144 0.468748 0.476562 0.484374 0.5 0.515626 0.523438 0.531252 0.546856 0.55467 0.56248 0.570293 0.578102 0.585915 0.593728 0.609339 0.624966 0.687472 0.749977 0.812483 0.874989 0.937494 1 1 1 1 projected
  arc A73 (541.0931, -463.5455) -> (547.6326, -455.8013) centre (0, 0) ccw projected
  spline S70 degree 3 poles (547.6326, -455.8013) (546.9825, -454.5712) (545.6823, -452.1111) (543.6571, -448.4612) (541.5755, -444.8434) (539.434, -441.2605) (537.2158, -437.725) (535.5364, -435.0826) (534.3423, -433.3707) (533.9201, -432.6078) (533.6585, -431.9619) (533.5296, -431.4557) (533.4301, -430.9425) (533.41, -430.42) (533.4272, -429.8979) (533.5398, -429.2102) (533.7712, -428.5479) (534.1023, -427.9349) (534.5159, -427.374) (535.0713, -426.7051) (535.5998, -426.0148) (536.0546, -425.4868) (536.5786, -425.0276) (537.1728, -424.6546) (537.8181, -424.3918) (538.3233, -424.2589) (538.8372, -424.1622) (539.3597, -424.1449) (539.8819, -424.158) (540.5699, -424.2693) (541.4076, -424.5112) (543.3422, -425.2944) (546.2921, -426.3437) (550.2325, -427.7196) (554.2022, -429.0101) (558.1924, -430.2345) (562.2015, -431.3967) (564.8892, -432.1169) (566.2331, -432.4769) knots 0 0 0 0 0.062506 0.125011 0.187517 0.250023 0.312528 0.375034 0.390661 0.406272 0.414085 0.421898 0.429707 0.43752 0.44533 0.453144 0.468748 0.476562 0.484374 0.5 0.515626 0.523438 0.531252 0.546856 0.55467 0.56248 0.570293 0.578102 0.585915 0.593728 0.609339 0.624966 0.687472 0.749977 0.812483 0.874989 0.937494 1 1 1 1 projected
  arc A74 (566.2331, -432.4769) -> (572.328, -424.3782) centre (0, 0) ccw projected
  spline S71 degree 3 poles (572.328, -424.3782) (571.61, -423.1866) (570.1739, -420.8032) (567.9472, -417.2726) (565.6661, -413.7772) (563.327, -410.32) (560.9141, -406.9145) (559.0892, -404.3703) (557.801, -402.7281) (557.3367, -401.9901) (557.0392, -401.3599) (556.8821, -400.8617) (556.7541, -400.3549) (556.7047, -399.8343) (556.6926, -399.312) (556.7665, -398.6191) (556.9604, -397.945) (557.2566, -397.3143) (557.638, -396.7311) (558.1551, -396.0322) (558.644, -395.3133) (559.0685, -394.7606) (559.566, -394.2727) (560.1383, -393.8671) (560.7679, -393.5684) (561.2648, -393.4074) (561.7725, -393.2821) (562.2931, -393.2355) (562.8153, -393.2193) (563.5084, -393.2919) (564.3583, -393.4864) (566.3339, -394.1599) (569.338, -395.0422) (573.3493, -396.1949) (577.3851, -397.2608) (581.4377, -398.2595) (585.5056, -399.1951) (588.2295, -399.7635) (589.5915, -400.0476) knots 0 0 0 0 0.062506 0.125011 0.187517 0.250023 0.312528 0.375034 0.390661 0.406272 0.414085 0.421898 0.429707 0.43752 0.44533 0.453144 0.468748 0.476562 0.484374 0.5 0.515626 0.523438 0.531252 0.546856 0.55467 0.56248 0.570293 0.578102 0.585915 0.593728 0.609339 0.624966 0.687472 0.749977 0.812483 0.874989 0.937494 1 1 1 1 projected
  arc A75 (589.5915, -400.0476) -> (595.2227, -391.6199) centre (0, 0) ccw projected
  spline S72 degree 3 poles (595.2227, -391.6199) (594.439, -390.4704) (592.8715, -388.1713) (590.4504, -384.7711) (587.9769, -381.4091) (585.4477, -378.0885) (582.8476, -374.8236) (580.8828, -372.3858) (579.5046, -370.8184) (578.9997, -370.1076) (578.6673, -369.495) (578.4825, -369.0064) (578.3263, -368.5076) (578.2478, -367.9906) (578.2064, -367.4699) (578.2414, -366.7739) (578.3971, -366.0899) (578.6575, -365.4436) (579.0056, -364.8399) (579.4827, -364.1131) (579.9306, -363.3679) (580.3234, -362.7924) (580.7927, -362.2774) (581.3414, -361.8402) (581.9532, -361.5068) (582.4404, -361.3181) (582.9402, -361.1645) (583.4575, -361.0889) (583.9779, -361.0434) (584.674, -361.077) (585.5335, -361.2235) (587.5436, -361.7852) (590.5925, -362.4976) (594.6622, -363.4237) (598.7514, -364.2616) (602.8536, -365.0315) (606.9676, -365.7376) (609.7191, -366.1523) (611.0948, -366.3596) knots 0 0 0 0 0.062506 0.125011 0.187517 0.250023 0.312528 0.375034 0.390661 0.406272 0.414085 0.421898 0.429707 0.43752 0.44533 0.453144 0.468748 0.476562 0.484374 0.5 0.515626 0.523438 0.531252 0.546856 0.55467 0.56248 0.570293 0.578102 0.585915 0.593728 0.609339 0.624966 0.687472 0.749977 0.812483 0.874989 0.937494 1 1 1 1 projected
  arc A76 (611.0948, -366.3596) -> (616.2446, -357.6294) centre (0, 0) ccw projected